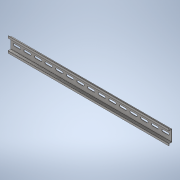
# Autodesk Inventor part: Riel 35x7.5 378mm
Saved by Autodesk Inventor 2021 (Build 250183000, 183)
## iProperties
Created: 2021-04-16
Part Number: Riel 35x7.5 378mm
Material: Steel, Galvanized
Document SubType Name: Modeling
Designer: Nelson
Density: 7.85 g/cm^3
Appearance: Galvanized
Mass: 132.092 g
Surface Area: 344.862 cm^2
Volume: 16.827 cm^3
Author: Nelson
Autodesk Inventor part; units mm, degrees
ref_plane "YZ Plane" through (0, 0, 0) normal (1, 0, 0) x (0, 1, 0)
ref_plane "XZ Plane" through (0, 0, 0) normal (0, 1, 0) x (-1, 0, 0)
ref_plane "XY Plane" through (0, 0, 0) normal (0, 0, 1) x (1, 0, 0)
sketch "Boceto principal" plane through (0, 0, 0) normal (1, 0, 0) x (0, 1, 0)
  line L0 (0, 0) -> (0, -1)
  line L1 (0, -1) -> (3.5, -1)
  line L2 (4, -1.5) -> (4, -7)
  line L3 (4.5, -7.5) -> (30.5, -7.5)
  line L4 (31, -7) -> (31, -1.5)
  line L5 (31.5, -1) -> (35, -1)
  line L6 (35, -1) -> (35, 0)
  line L7 (35, 0) -> (30.5, 0)
  line L8 (30, -0.5) -> (30, -6)
  line L9 (29.5, -6.5) -> (5.5, -6.5)
  line L10 (5, -6) -> (5, -0.5)
  line L11 (4.5, 0) -> (0, 0)
  arc A0 (4, -1.5) -> (3.5, -1) centre (3.5, -1.5) ccw
  arc A1 (4, -7) -> (4.5, -7.5) centre (4.5, -7) ccw
  arc A2 (30.5, -7.5) -> (31, -7) centre (30.5, -7) ccw
  arc A3 (31.5, -1) -> (31, -1.5) centre (31.5, -1.5) ccw
  arc A4 (30.5, 0) -> (30, -0.5) centre (30.5, -0.5) ccw
  arc A5 (29.5, -6.5) -> (30, -6) centre (29.5, -6) ccw
  arc A6 (5, -6) -> (5.5, -6.5) centre (5.5, -6) ccw
  arc A7 (5, -0.5) -> (4.5, 0) centre (4.5, -0.5) ccw
  constraints: 24 end point, 16 point on circle, 8 centre point
extrude "Extrusion1" add sketch "Boceto principal" along normal blind 378
sketch "Boceto agujeros" plane through (0, 0, 0) normal (0, 0, 1) x (1, 0, 0)
  line L0 (7.6, 14.9) -> (20.4, 14.9)
  line L1 (20.4, 20.1) -> (7.6, 20.1)
  arc A0 (7.6, 20.1) -> (7.6, 14.9) centre (7.6, 17.5) ccw
  arc A1 (20.4, 14.9) -> (20.4, 20.1) centre (20.4, 17.5) ccw
  constraints: 4 end point, 4 point on circle, 2 centre point
extrude "Extrusion2" cut sketch "Boceto agujeros" against normal blind 15
pattern_linear "Rectangular Pattern1" count 16 spacing 25 along (1, 0, 0) of "Extrusion2"
body "Solid1"
